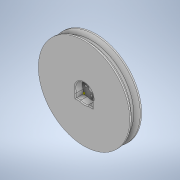
# Autodesk Inventor part: s_base7
Saved by Autodesk Inventor 2022 (Build 260153000, 153)
## iProperties
Created: 2021-09-15
Part Number: s_base7
Material: Generic
Document SubType Name: Modeling
Designer: yuto6
Density: 1 g/cm^3
Appearance: Default
Author: yuto6
Autodesk Inventor part; units mm, degrees
ref_plane "YZ Plane" through (0, 0, 0) normal (1, 0, 0) x (0, 1, 0)
ref_plane "XZ Plane" through (0, 0, 0) normal (0, 1, 0) x (-1, 0, 0)
ref_plane "XY Plane" through (0, 0, 0) normal (0, 0, 1) x (1, 0, 0)
sketch "スケッチ1" plane through (0, 0, 0) normal (1, 0, 0) x (0, 1, 0)
  line L0 (0, 0) -> (0, -10)
  line L1 (0, 0) -> (50, 0)
  line L2 (0, -10) -> (50, -10)
  line L3 (50, 0) -> (40, -10)
  line L4 (50, -10) -> (40, 0)
  circle A0 centre (47.8284, -5) radius 2
  line L5 (0, 0) -> (50, 0)
  line L6 (50, 0) -> (50, 1.5)
  line L7 (50, 1.5) -> (0, 1.5)
  line L8 (0, 1.5) -> (0, 0)
  line L9 (0, -10) -> (50, -10)
  line L10 (50, -10) -> (50, -11.5)
  line L11 (50, -11.5) -> (0, -11.5)
  line L12 (0, -11.5) -> (0, -10)
  point P0 (46.4142, -6.4142)
  point P1 (46.4142, -3.5858)
  dimension "d0" = 10
  dimension "d1" = 50
  dimension "d2" = 50
  dimension "d3" = 45
  dimension "d4" = 45
  dimension "d5" = 2
  dimension "d6" = 2
  dimension "d7" = 1.5
  dimension "d8" = 1.5
  dimension "d41" = 50
  constraints: 26 end point, 4 horizontal, 4 parallel, 3 point on line, 2 perpendicular, 1 centre point, 1 tangent, 1 vertical
  measures "d0" distance of L0.start L0.end
  measures "d1" distance of L0.start L1.end
  measures "d2" distance of L0.end L2.end
  measures "d3" angle of L1 L3
  measures "d4" angle of L2 L4
  measures "d5" distance from line of L3 A0.centre
  measures "d6" distance from line of L4 A0.centre
  measures "d7" distance between parallel lines of L5 L7
  measures "d8" distance between parallel lines of L2 L11
  measures "d41" distance between parallel lines of L8 L6
revolve "回転1" add sketch "スケッチ1" angle 360 about axis through (0, 0, 0) along (0, 0, -1) contours L1 L4 L3 L2 L0 | L8 L7 L6 L1 | L2 L10 L11 L12 | L1 L3 L4 | L3 L4 L2 | L3 A0 L4
sketch "スケッチ2" plane through (0, 0, 1.5) normal (0, 0, 1) x (1, 0, 0)
  point P0 (0, 0)
  point P1 (0, 0)
  constraints: 1 coincident
hole "穴1" at (0, 0, 1.5) direction (0, 0, -1) diameter 6.5 end through all
sketch "スケッチ3" plane through (0, 0, 1.5) normal (0, 0, 1) x (1, 0, 0)
  circle A0 centre (0, 0) radius 10
  line L0 (-9, 0) -> (9, 0)
  line L1 (9, 0) -> (9, -9)
  line L2 (9, -9) -> (-9, -9)
  line L3 (-9, -9) -> (-9, 0)
  point P0 (0, 0)
  point P1 (4.3589, -9)
  point P2 (9, -4.3589)
  point P3 (-9, -4.3589)
  point P4 (-4.3589, -9)
  dimension "d17" = 20
  dimension "d36" = 18
  dimension "d37" = 9
  dimension "d38" = 9
  dimension "d39" = 0
  constraints: 8 end point, 2 parallel, 1 centre point, 1 coincident, 1 horizontal, 1 perpendicular
  measures "d17" diameter of A0
  measures "d36" distance between parallel lines of L1 L3
  measures "d37" distance from line of point (0, 0) L3
  measures "d38" distance between parallel lines of L2 L0
  measures "d39" distance from line of point (0, 0) L0
extrude "押し出し1" cut sketch "スケッチ3" against normal blind 8
sketch "スケッチ4" plane through (0, 0, 1.5) normal (0, 0, 1) x (1, 0, 0)
  point P0 (0, 0)
sketch "スケッチ5" plane through (0, 0, -11.5) normal (0, 0, -1) x (-1, 0, 0)
  circle A0 centre (0, 0) radius 6
  point P0 (0, 0)
  point P1 (6, 0)
  point P2 (0, 6)
  point P3 (-6, 0)
  point P4 (0, -6)
  dimension "d20" = 12
  dimension "d23" = 360
  constraints: 1 coincident, 1 horizontal alignment, 7 other
hole "穴2" at (-6, 0, -11.5) at (0, 6, -11.5) at (6, 0, -11.5) at (0, -6, -11.5) direction (0, 0, 1) diameter 2.5 end through all
fillet "フィレット2" radius 1 6 edges at (0, 10, 1.5) (-9, -6.6794, 1.5) (-6.6794, -9, 1.5) (0, -10, 1.5) (6.6794, -9, 1.5) (9, -6.6794, 1.5)
equation "\"d2\" = d1"
equation "\"d6\" = d5"
equation "\"d8\" = d7"
equation "\"d41\" = d1"
equation "\"d37\" = 0.5 * d36"
